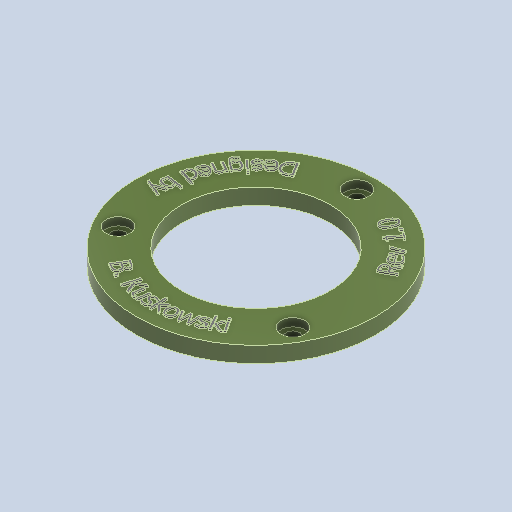
# Autodesk Inventor part: name_plate
Saved by Autodesk Inventor 2025 (Build 290162000, 162)
## iProperties
Created: 2026-08-15
Part Number: name_plate
Material: Ogólny
Document SubType Name: Modeling
Designer: zzapa
Density: 1 g/cm^3
Appearance: Ciemnooliwkowa
Author: zzapa
Autodesk Inventor part; units mm, degrees
ref_plane "YZ Plane" through (0, 0, 0) normal (1, 0, 0) x (0, 1, 0)
ref_plane "XZ Plane" through (0, 0, 0) normal (0, 1, 0) x (-1, 0, 0)
ref_plane "XY Plane" through (0, 0, 0) normal (0, 0, 1) x (1, 0, 0)
sketch "Szkic1" plane through (0, 0, 0) normal (0, 1, 0) x (-1, 0, 0)
  circle A0 centre (0, 0) radius 14
  circle A1 centre (0, 0) radius 22.5
  dimension "d13" = 28
  dimension "d14" = 45
  constraints: 2 centre point, 2 coincident
  measures "d13" diameter of A0
  measures "d14" diameter of A1
extrude "Wyciągnięcie proste1" add sketch "Szkic1" along normal blind 3
sketch "Szkic2" plane through (0, 3, 0) normal (0, 1, 0) x (1, 0, 0)
  line L0 (0, 31.5) -> (0, -31.5) projected
  point P0 (0, 0)
  point P1 (0, 19)
  point P2 (-16.4545, -9.5)
  point P3 (16.4545, -9.5)
  dimension "d4" = 360
  dimension "d15" = 19
  constraints: 1 point on line, 4 other
  measures "d15" distance of point (0, 0) point (0, 19)
hole "Otwór1" at (0, 3, -19) at (-16.4545, 3, 9.5) at (16.4545, 3, 9.5) direction (0, -1, 0) diameter 2.6 end through all counterbore diameter 4.5 counterbore depth 1.5
sketch "Szkic3" plane through (0, 3, 0) normal (0, 1, 0) x (1, 0, 0)
  circle A0 centre (0, 0) radius 14 projected
  circle A1 centre (0, 0) radius 22.5 projected
  circle A2 centre (0, 0) radius 14 projected
  line L0 (0, -14) -> (0, -22.5)
  line L1 (0, 31.5) -> (0, -31.5) projected
  circle A3 centre (0, 0) radius 20
  spline S0 degree 2 poles (-10.7525, 15.0832) (-10.9705, 15.4392) (-11.0329, 16.1888) (-10.8887, 16.4973) knots 0 0 0 1 2 2 2
  spline S1 degree 2 poles (-10.8887, 16.4973) (-10.7669, 16.7428) (-10.412, 17.0761) (-10.096, 17.2696) knots 0 0 0 1 2 2 2
  line L2 (-10.096, 17.2696) -> (-9.4978, 17.636)
  line L3 (-9.4978, 17.636) -> (-7.9058, 15.0369)
  line L4 (-7.9058, 15.0369) -> (-8.4976, 14.6743)
  spline S2 degree 2 poles (-8.4976, 14.6743) (-8.8641, 14.4498) (-9.3483, 14.3039) (-9.555, 14.3105) knots 0 0 0 1 2 2 2
  spline S3 degree 2 poles (-9.555, 14.3105) (-9.9076, 14.3234) (-10.5203, 14.7041) (-10.7525, 15.0832) knots 0 0 0 1 2 2 2
  spline S4 degree 2 poles (-10.3897, 15.2996) (-10.2065, 15.0005) (-9.7492, 14.6984) (-9.4798, 14.6984) knots 0 0 0 1 2 2 2
  spline S5 degree 2 poles (-9.4798, 14.6984) (-9.2905, 14.7014) (-8.9315, 14.8199) (-8.6977, 14.9631) knots 0 0 0 1 2 2 2
  line L5 (-8.6977, 14.9631) -> (-8.4344, 15.1244)
  line L6 (-8.4344, 15.1244) -> (-9.6601, 17.1253)
  line L7 (-9.6601, 17.1253) -> (-9.9234, 16.9641)
  spline S6 degree 2 poles (-9.9234, 16.9641) (-10.1529, 16.8234) (-10.4553, 16.5368) (-10.5358, 16.3514) knots 0 0 0 1 2 2 2
  spline S7 degree 2 poles (-10.5358, 16.3514) (-10.6421, 16.1183) (-10.5755, 15.6029) (-10.3897, 15.2996) knots 0 0 0 1 2 2 2
  spline S8 degree 2 poles (-12.6723, 15.5409) (-12.2444, 15.8838) (-11.3895, 15.7808) (-11.0342, 15.3375) knots 0 0 0 1 2 2 2
  spline S9 degree 2 poles (-11.0342, 15.3375) (-10.6851, 14.9019) (-10.7279, 14.0193) (-11.096, 13.7243) knots 0 0 0 1 2 2 2
  spline S10 degree 2 poles (-11.096, 13.7243) (-11.2618, 13.5914) (-11.5953, 13.4823) (-11.7716, 13.5088) knots 0 0 0 1 2 2 2
  spline S11 degree 2 poles (-11.7716, 13.5088) (-11.9499, 13.5337) (-12.2884, 13.7467) (-12.4598, 13.9607) knots 0 0 0 1 2 2 2
  line L8 (-12.4598, 13.9607) -> (-12.5911, 14.1245)
  line L9 (-12.5911, 14.1245) -> (-11.3557, 15.1147)
  spline S12 degree 2 poles (-11.3557, 15.1147) (-11.6044, 15.425) (-12.1808, 15.5043) (-12.4583, 15.2819) knots 0 0 0 1 2 2 2
  spline S13 degree 2 poles (-12.4583, 15.2819) (-12.5566, 15.2031) (-12.7119, 15.0058) (-12.7612, 14.9094) knots 0 0 0 1 2 2 2
  spline S14 degree 2 poles (-12.7612, 14.9094) (-12.8112, 14.8059) (-12.869, 14.6489) (-12.8809, 14.5887) knots 0 0 0 1 2 2 2
  line L10 (-12.8809, 14.5887) -> (-12.8982, 14.5748)
  line L11 (-12.8982, 14.5748) -> (-13.1608, 14.9024)
  spline S15 degree 2 poles (-13.1608, 14.9024) (-13.1258, 14.9654) (-13.0172, 15.1537) (-12.9694, 15.2205) knots 0 0 0 1 2 2 2
  spline S16 degree 2 poles (-12.9694, 15.2205) (-12.9027, 15.315) (-12.7802, 15.4544) (-12.6723, 15.5409) knots 0 0 0 1 2 2 2
  spline S17 degree 2 poles (-12.1144, 14.1299) (-12.0132, 14.0116) (-11.821, 13.8745) (-11.7249, 13.8533) knots 0 0 0 1 2 2 2
  spline S18 degree 2 poles (-11.7249, 13.8533) (-11.6188, 13.8276) (-11.3978, 13.8876) (-11.2764, 13.9849) knots 0 0 0 1 2 2 2
  spline S19 degree 2 poles (-11.2764, 13.9849) (-11.1569, 14.0806) (-11.0464, 14.2864) (-11.0326, 14.4113) knots 0 0 0 1 2 2 2
  spline S20 degree 2 poles (-11.0326, 14.4113) (-11.0223, 14.5367) (-11.0904, 14.7639) (-11.1719, 14.8853) knots 0 0 0 1 2 2 2
  line L12 (-11.1719, 14.8853) -> (-12.1144, 14.1299)
  spline S21 degree 2 poles (-14.0398, 14.32) (-13.8761, 14.4811) (-13.506, 14.672) (-13.3642, 14.7146) knots 0 0 0 1 2 2 2
  line L13 (-13.3642, 14.7146) -> (-13.061, 14.4065)
  line L14 (-13.061, 14.4065) -> (-13.0751, 14.3926)
  spline S22 degree 2 poles (-13.0751, 14.3926) (-13.138, 14.3861) (-13.2989, 14.3595) (-13.4145, 14.3185) knots 0 0 0 1 2 2 2
  spline S23 degree 2 poles (-13.4145, 14.3185) (-13.5161, 14.2844) (-13.7336, 14.1673) (-13.8234, 14.079) knots 0 0 0 1 2 2 2
  spline S24 degree 2 poles (-13.8234, 14.079) (-13.8885, 14.0148) (-14.0087, 13.8377) (-14.0197, 13.7784) knots 0 0 0 1 2 2 2
  spline S25 degree 2 poles (-14.0197, 13.7784) (-14.0378, 13.6947) (-14.0091, 13.5739) (-13.9329, 13.4965) knots 0 0 0 1 2 2 2
  spline S26 degree 2 poles (-13.9329, 13.4965) (-13.8376, 13.3996) (-13.6332, 13.4032) (-13.4647, 13.5032) knots 0 0 0 1 2 2 2
  spline S27 degree 2 poles (-13.4647, 13.5032) (-13.3998, 13.5429) (-13.1961, 13.674) (-13.1049, 13.7257) knots 0 0 0 1 2 2 2
  spline S28 degree 2 poles (-13.1049, 13.7257) (-12.8646, 13.8547) (-12.4738, 13.7957) (-12.3161, 13.6355) knots 0 0 0 1 2 2 2
  spline S29 degree 2 poles (-12.3161, 13.6355) (-12.0978, 13.4137) (-12.1585, 12.8099) (-12.4331, 12.5396) knots 0 0 0 1 2 2 2
  spline S30 degree 2 poles (-12.4331, 12.5396) (-12.5687, 12.4062) (-12.9092, 12.2028) (-13.0527, 12.162) knots 0 0 0 1 2 2 2
  line L15 (-13.0527, 12.162) -> (-13.3421, 12.456)
  line L16 (-13.3421, 12.456) -> (-13.328, 12.4699)
  spline S31 degree 2 poles (-13.328, 12.4699) (-13.1392, 12.4893) (-12.7869, 12.6455) (-12.6548, 12.7754) knots 0 0 0 1 2 2 2
  spline S32 degree 2 poles (-12.6548, 12.7754) (-12.5193, 12.9088) (-12.4453, 13.2069) (-12.5579, 13.3213) knots 0 0 0 1 2 2 2
  spline S33 degree 2 poles (-12.5579, 13.3213) (-12.6601, 13.4252) (-12.8698, 13.4164) (-13.0242, 13.3268) knots 0 0 0 1 2 2 2
  spline S34 degree 2 poles (-13.0242, 13.3268) (-13.0997, 13.2837) (-13.2822, 13.1664) (-13.384, 13.1043) knots 0 0 0 1 2 2 2
  spline S35 degree 2 poles (-13.384, 13.1043) (-13.6087, 12.9734) (-13.9979, 13.0027) (-14.1764, 13.184) knots 0 0 0 1 2 2 2
  spline S36 degree 2 poles (-14.1764, 13.184) (-14.2803, 13.2896) (-14.3812, 13.5577) (-14.3678, 13.706) knots 0 0 0 1 2 2 2
  spline S37 degree 2 poles (-14.3678, 13.706) (-14.3526, 13.8631) (-14.2071, 14.1554) (-14.0398, 14.32) knots 0 0 0 1 2 2 2
  line L17 (-15.1279, 13.0838) -> (-14.873, 13.3728)
  line L18 (-14.873, 13.3728) -> (-13.1575, 11.86)
  line L19 (-13.1575, 11.86) -> (-13.4124, 11.571)
  line L20 (-13.4124, 11.571) -> (-15.1279, 13.0838)
  line L21 (-13.1451, 11.299) -> (-12.8559, 11.6269)
  line L22 (-12.8559, 11.6269) -> (-12.5558, 11.3622)
  line L23 (-12.5558, 11.3622) -> (-12.8449, 11.0343)
  line L24 (-12.8449, 11.0343) -> (-13.1451, 11.299)
  spline S38 degree 2 poles (-15.8473, 12.8162) (-15.8848, 12.7949) (-16.0184, 12.7066) (-16.0938, 12.6427) knots 0 0 0 1 2 2 2
  spline S39 degree 2 poles (-16.0938, 12.6427) (-16.1791, 12.5738) (-16.3127, 12.4485) (-16.3762, 12.3633) knots 0 0 0 1 2 2 2
  spline S40 degree 2 poles (-16.3762, 12.3633) (-16.4825, 12.2208) (-16.555, 11.9667) (-16.529, 11.861) knots 0 0 0 1 2 2 2
  spline S41 degree 2 poles (-16.529, 11.861) (-16.5015, 11.7574) (-16.3564, 11.5844) (-16.2435, 11.5002) knots 0 0 0 1 2 2 2
  line L25 (-16.2435, 11.5002) -> (-16.0831, 11.3805)
  spline S42 degree 2 poles (-16.0831, 11.3805) (-16.099, 11.5865) (-16.0232, 11.9029) (-15.8888, 12.083) knots 0 0 0 1 2 2 2
  spline S43 degree 2 poles (-15.8888, 12.083) (-15.6555, 12.3959) (-14.9141, 12.419) (-14.4765, 12.0927) knots 0 0 0 1 2 2 2
  spline S44 degree 2 poles (-14.4765, 12.0927) (-14.2488, 11.9228) (-13.9924, 11.5312) (-13.9474, 11.3313) knots 0 0 0 1 2 2 2
  spline S45 degree 2 poles (-13.9474, 11.3313) (-13.9074, 11.1412) (-13.9899, 10.7621) (-14.1021, 10.6116) knots 0 0 0 1 2 2 2
  spline S46 degree 2 poles (-14.1021, 10.6116) (-14.2085, 10.4691) (-14.4309, 10.3114) (-14.5705, 10.2522) knots 0 0 0 1 2 2 2
  line L26 (-14.5705, 10.2522) -> (-14.5066, 10.1768)
  line L27 (-14.5066, 10.1768) -> (-14.7237, 9.8858)
  line L28 (-14.7237, 9.8858) -> (-16.3472, 11.0968)
  spline S47 degree 2 poles (-16.3472, 11.0968) (-16.8144, 11.4453) (-16.9472, 12.1761) (-16.6356, 12.5939) knots 0 0 0 1 2 2 2
  spline S48 degree 2 poles (-16.6356, 12.5939) (-16.5352, 12.7285) (-16.2819, 12.9771) (-16.1562, 13.0713) knots 0 0 0 1 2 2 2
  line L29 (-16.1562, 13.0713) -> (-15.8355, 12.8321)
  line L30 (-15.8355, 12.8321) -> (-15.8473, 12.8162)
  line L31 (-15.8297, 11.1915) -> (-14.8219, 10.4398)
  spline S49 degree 2 poles (-14.8219, 10.4398) (-14.6809, 10.5133) (-14.4886, 10.6719) (-14.4162, 10.7689) knots 0 0 0 1 2 2 2
  spline S50 degree 2 poles (-14.4162, 10.7689) (-14.242, 11.0025) (-14.3856, 11.5287) (-14.7083, 11.7695) knots 0 0 0 1 2 2 2
  spline S51 degree 2 poles (-14.7083, 11.7695) (-15.0132, 11.9969) (-15.4841, 12.0307) (-15.6554, 11.8011) knots 0 0 0 1 2 2 2
  spline S52 degree 2 poles (-15.6554, 11.8011) (-15.7455, 11.6803) (-15.8395, 11.356) (-15.8297, 11.1915) knots 0 0 0 1 2 2 2
  line L32 (-17.7638, 9.2342) -> (-17.5707, 9.5677)
  line L33 (-17.5707, 9.5677) -> (-16.442, 8.9144)
  spline S53 degree 2 poles (-16.442, 8.9144) (-16.3052, 8.8352) (-16.0552, 8.7248) (-15.9624, 8.7224) knots 0 0 0 1 2 2 2
  spline S54 degree 2 poles (-15.9624, 8.7224) (-15.864, 8.7197) (-15.7072, 8.823) (-15.6354, 8.947) knots 0 0 0 1 2 2 2
  spline S55 degree 2 poles (-15.6354, 8.947) (-15.5637, 9.071) (-15.544, 9.4106) (-15.5779, 9.5986) knots 0 0 0 1 2 2 2
  line L34 (-15.5779, 9.5986) -> (-17.0572, 10.4549)
  line L35 (-17.0572, 10.4549) -> (-16.8642, 10.7884)
  line L36 (-16.8642, 10.7884) -> (-14.8847, 9.6426)
  line L37 (-14.8847, 9.6426) -> (-15.0777, 9.3091)
  line L38 (-15.0777, 9.3091) -> (-15.2979, 9.4366)
  spline S56 degree 2 poles (-15.2979, 9.4366) (-15.2498, 9.209) (-15.2758, 8.8387) (-15.3698, 8.6762) knots 0 0 0 1 2 2 2
  spline S57 degree 2 poles (-15.3698, 8.6762) (-15.5381, 8.3855) (-16.1134, 8.279) (-16.479, 8.4906) knots 0 0 0 1 2 2 2
  line L39 (-16.479, 8.4906) -> (-17.7638, 9.2342)
  spline S58 degree 2 poles (-18.4477, 7.8607) (-18.2285, 8.3633) (-17.4238, 8.6699) (-16.903, 8.4428) knots 0 0 0 1 2 2 2
  spline S59 degree 2 poles (-16.903, 8.4428) (-16.3914, 8.2196) (-16.0186, 7.4184) (-16.2072, 6.986) knots 0 0 0 1 2 2 2
  spline S60 degree 2 poles (-16.2072, 6.986) (-16.2921, 6.7913) (-16.5366, 6.5395) (-16.705, 6.4809) knots 0 0 0 1 2 2 2
  spline S61 degree 2 poles (-16.705, 6.4809) (-16.8744, 6.42) (-17.2731, 6.4511) (-17.5244, 6.5607) knots 0 0 0 1 2 2 2
  line L40 (-17.5244, 6.5607) -> (-17.7169, 6.6446)
  line L41 (-17.7169, 6.6446) -> (-17.0839, 8.0959)
  spline S62 degree 2 poles (-17.0839, 8.0959) (-17.4485, 8.2549) (-17.9956, 8.0569) (-18.1378, 7.7309) knots 0 0 0 1 2 2 2
  spline S63 degree 2 poles (-18.1378, 7.7309) (-18.1881, 7.6155) (-18.2338, 7.3686) (-18.2325, 7.2603) knots 0 0 0 1 2 2 2
  spline S64 degree 2 poles (-18.2325, 7.2603) (-18.2287, 7.1454) (-18.2068, 6.9796) (-18.1893, 6.9207) knots 0 0 0 1 2 2 2
  line L42 (-18.1893, 6.9207) -> (-18.1982, 6.9004)
  line L43 (-18.1982, 6.9004) -> (-18.5831, 7.0682)
  spline S65 degree 2 poles (-18.5831, 7.0682) (-18.5813, 7.1402) (-18.5728, 7.3575) (-18.5616, 7.4388) knots 0 0 0 1 2 2 2
  spline S66 degree 2 poles (-18.5616, 7.4388) (-18.5466, 7.5535) (-18.5029, 7.7339) (-18.4477, 7.8607) knots 0 0 0 1 2 2 2
  spline S67 degree 2 poles (-17.2974, 6.8713) (-17.1527, 6.8136) (-16.9188, 6.7816) (-16.8239, 6.8076) knots 0 0 0 1 2 2 2
  spline S68 degree 2 poles (-16.8239, 6.8076) (-16.718, 6.8342) (-16.5503, 6.9901) (-16.4881, 7.1327) knots 0 0 0 1 2 2 2
  spline S69 degree 2 poles (-16.4881, 7.1327) (-16.4269, 7.2731) (-16.4247, 7.5066) (-16.4707, 7.6237) knots 0 0 0 1 2 2 2
  spline S70 degree 2 poles (-16.4707, 7.6237) (-16.5199, 7.7395) (-16.6859, 7.9088) (-16.8145, 7.9784) knots 0 0 0 1 2 2 2
  line L44 (-16.8145, 7.9784) -> (-17.2974, 6.8713)
  line L45 (-19.3752, 5.0374) -> (-19.2619, 5.4058)
  line L46 (-19.2619, 5.4058) -> (-19.04, 5.3375)
  spline S71 degree 2 poles (-19.04, 5.3375) (-19.0847, 5.4443) (-19.1407, 5.5985) (-19.1547, 5.6958) knots 0 0 0 1 2 2 2
  spline S72 degree 2 poles (-19.1547, 5.6958) (-19.1685, 5.7853) (-19.1571, 5.9653) (-19.123, 6.0762) knots 0 0 0 1 2 2 2
  spline S73 degree 2 poles (-19.123, 6.0762) (-19.0678, 6.2557) (-18.8261, 6.5121) (-18.6494, 6.5741) knots 0 0 0 1 2 2 2
  spline S74 degree 2 poles (-18.6494, 6.5741) (-18.4728, 6.6361) (-18.0115, 6.6234) (-17.7353, 6.5385) knots 0 0 0 1 2 2 2
  spline S75 degree 2 poles (-17.7353, 6.5385) (-17.4472, 6.4499) (-17.0727, 6.172) (-16.9545, 5.9935) knots 0 0 0 1 2 2 2
  spline S76 degree 2 poles (-16.9545, 5.9935) (-16.8498, 5.8295) (-16.7907, 5.4418) (-16.8481, 5.2553) knots 0 0 0 1 2 2 2
  spline S77 degree 2 poles (-16.8481, 5.2553) (-16.8982, 5.0924) (-17.0461, 4.8717) (-17.1631, 4.7604) knots 0 0 0 1 2 2 2
  line L47 (-17.1631, 4.7604) -> (-16.2187, 4.47)
  line L48 (-16.2187, 4.47) -> (-16.3319, 4.1017)
  line L49 (-16.3319, 4.1017) -> (-19.3752, 5.0374)
  line L50 (-18.7307, 5.2424) -> (-17.4676, 4.854)
  spline S78 degree 2 poles (-17.4676, 4.854) (-17.3594, 4.9707) (-17.243, 5.1726) (-17.2046, 5.2977) knots 0 0 0 1 2 2 2
  spline S79 degree 2 poles (-17.2046, 5.2977) (-17.1175, 5.5811) (-17.4437, 6.0328) (-17.8451, 6.1562) knots 0 0 0 1 2 2 2
  spline S80 degree 2 poles (-17.8451, 6.1562) (-18.2323, 6.2753) (-18.7162, 6.1553) (-18.7997, 5.8838) knots 0 0 0 1 2 2 2
  spline S81 degree 2 poles (-18.7997, 5.8838) (-18.844, 5.7398) (-18.8018, 5.4064) (-18.7307, 5.2424) knots 0 0 0 1 2 2 2
  spline S82 degree 2 poles (-18.8116, 1.1694) (-19.3684, 1.235) (-19.9844, 1.8546) (-19.9365, 2.2618) knots 0 0 0 1 2 2 2
  spline S83 degree 2 poles (-19.9365, 2.2618) (-19.9148, 2.4458) (-19.7932, 2.6976) (-19.6997, 2.8159) knots 0 0 0 1 2 2 2
  line L51 (-19.6997, 2.8159) -> (-19.8023, 2.8529)
  line L52 (-19.8023, 2.8529) -> (-19.7601, 3.211)
  line L53 (-19.7601, 3.211) -> (-16.5981, 2.8389)
  line L54 (-16.5981, 2.8389) -> (-16.6431, 2.4562)
  line L55 (-16.6431, 2.4562) -> (-17.7716, 2.589)
  spline S84 degree 2 poles (-17.7716, 2.589) (-17.6586, 2.429) (-17.5264, 2.0727) (-17.5515, 1.8593) knots 0 0 0 1 2 2 2
  spline S85 degree 2 poles (-17.5515, 1.8593) (-17.5969, 1.4741) (-18.2646, 1.1051) (-18.8116, 1.1694) knots 0 0 0 1 2 2 2
  spline S86 degree 2 poles (-18.7945, 1.5679) (-18.3873, 1.5199) (-17.9362, 1.718) (-17.9039, 1.9928) knots 0 0 0 1 2 2 2
  spline S87 degree 2 poles (-17.9039, 1.9928) (-17.8857, 2.1473) (-17.9954, 2.4835) (-18.0929, 2.6268) knots 0 0 0 1 2 2 2
  line L56 (-18.0929, 2.6268) -> (-19.3955, 2.7801)
  spline S88 degree 2 poles (-19.3955, 2.7801) (-19.4837, 2.6438) (-19.5688, 2.4275) (-19.5844, 2.295) knots 0 0 0 1 2 2 2
  spline S89 degree 2 poles (-19.5844, 2.295) (-19.6188, 2.0031) (-19.2435, 1.6207) (-18.7945, 1.5679) knots 0 0 0 1 2 2 2
  line L57 (-17.7197, -0.9043) -> (-20.8403, 0.3482)
  line L58 (-20.8403, 0.3482) -> (-20.8374, 0.7607)
  line L59 (-20.8374, 0.7607) -> (-19.8869, 0.3438)
  line L60 (-19.8869, 0.3438) -> (-17.7049, 1.1581)
  line L61 (-17.7049, 1.1581) -> (-17.7079, 0.7432)
  line L62 (-17.7079, 0.7432) -> (-19.4068, 0.1304)
  line L63 (-19.4068, 0.1304) -> (-17.7168, -0.5041)
  line L64 (-17.7168, -0.5041) -> (-17.7197, -0.9043)
  spline S90 degree 2 poles (-8.8291, -16.9346) (-8.946, -17.1294) (-9.2735, -17.3391) (-9.4548, -17.3629) knots 0 0 0 1 2 2 2
  spline S91 degree 2 poles (-9.4548, -17.3629) (-9.6717, -17.3883) (-10.0669, -17.2837) (-10.3338, -17.1236) knots 0 0 0 1 2 2 2
  line L65 (-10.3338, -17.1236) -> (-11.0836, -16.6737)
  line L66 (-11.0836, -16.6737) -> (-9.5155, -14.06)
  line L67 (-9.5155, -14.06) -> (-8.8229, -14.4755)
  spline S92 degree 2 poles (-8.8229, -14.4755) (-8.5433, -14.6433) (-8.2853, -14.847) (-8.2001, -14.9932) knots 0 0 0 1 2 2 2
  spline S93 degree 2 poles (-8.2001, -14.9932) (-8.1027, -15.1524) (-8.1196, -15.4735) (-8.2188, -15.6387) knots 0 0 0 1 2 2 2
  spline S94 degree 2 poles (-8.2188, -15.6387) (-8.3293, -15.823) (-8.6995, -15.9984) (-8.9207, -15.9781) knots 0 0 0 1 2 2 2
  line L68 (-8.9207, -15.9781) -> (-8.9283, -15.9908)
  spline S95 degree 2 poles (-8.9283, -15.9908) (-8.7334, -16.1941) (-8.6792, -16.6846) (-8.8291, -16.9346) knots 0 0 0 1 2 2 2
  spline S96 degree 2 poles (-9.2002, -16.7321) (-9.1113, -16.5838) (-9.0816, -16.3424) (-9.168, -16.1984) knots 0 0 0 1 2 2 2
  spline S97 degree 2 poles (-9.168, -16.1984) (-9.2252, -16.1064) (-9.4048, -15.9641) (-9.5849, -15.8561) knots 0 0 0 1 2 2 2
  line L69 (-9.5849, -15.8561) -> (-9.9788, -15.6197)
  line L70 (-9.9788, -15.6197) -> (-10.5583, -16.5856)
  line L71 (-10.5583, -16.5856) -> (-10.2766, -16.7546)
  spline S98 degree 2 poles (-10.2766, -16.7546) (-10.0478, -16.8918) (-9.7598, -17.007) (-9.6175, -17.0003) knots 0 0 0 1 2 2 2
  spline S99 degree 2 poles (-9.6175, -17.0003) (-9.4781, -16.9888) (-9.2828, -16.8698) (-9.2002, -16.7321) knots 0 0 0 1 2 2 2
  spline S100 degree 2 poles (-8.6102, -15.4702) (-8.5543, -15.377) (-8.5339, -15.1991) (-8.5797, -15.1169) knots 0 0 0 1 2 2 2
  spline S101 degree 2 poles (-8.5797, -15.1169) (-8.6365, -15.0194) (-8.8292, -14.875) (-9.0135, -14.7645) knots 0 0 0 1 2 2 2
  line L72 (-9.0135, -14.7645) -> (-9.346, -14.5649)
  line L73 (-9.346, -14.5649) -> (-9.8047, -15.3296)
  line L74 (-9.8047, -15.3296) -> (-9.4108, -15.5659)
  spline S102 degree 2 poles (-9.4108, -15.5659) (-9.2477, -15.6638) (-9.0727, -15.7226) (-8.9584, -15.7193) knots 0 0 0 1 2 2 2
  spline S103 degree 2 poles (-8.9584, -15.7193) (-8.8474, -15.7167) (-8.6839, -15.593) (-8.6102, -15.4702) knots 0 0 0 1 2 2 2
  line L75 (-8.4266, -18.1397) -> (-8.8676, -17.9284)
  line L76 (-8.8676, -17.9284) -> (-8.6157, -17.4027)
  line L77 (-8.6157, -17.4027) -> (-8.1747, -17.6141)
  line L78 (-8.1747, -17.6141) -> (-8.4266, -18.1397)
  line L79 (-4.4403, -19.5441) -> (-4.9447, -19.3945)
  line L80 (-4.9447, -19.3945) -> (-5.6096, -17.7185)
  line L81 (-5.6096, -17.7185) -> (-5.837, -17.8598)
  line L82 (-5.837, -17.8598) -> (-6.1832, -19.0273)
  line L83 (-6.1832, -19.0273) -> (-6.5716, -18.9121)
  line L84 (-6.5716, -18.9121) -> (-5.705, -15.9899)
  line L85 (-5.705, -15.9899) -> (-5.3167, -16.105)
  line L86 (-5.3167, -16.105) -> (-5.7148, -17.4478)
  line L87 (-5.7148, -17.4478) -> (-4.1184, -16.4604)
  line L88 (-4.1184, -16.4604) -> (-3.6448, -16.6008)
  line L89 (-3.6448, -16.6008) -> (-5.2418, -17.5468)
  line L90 (-5.2418, -17.5468) -> (-4.4403, -19.5441)
  line L91 (-2.4749, -19.8662) -> (-2.8548, -19.8016)
  line L92 (-2.8548, -19.8016) -> (-2.8126, -19.5532)
  spline S104 degree 2 poles (-2.8126, -19.5532) (-3.014, -19.6768) (-3.355, -19.7817) (-3.5498, -19.7486) knots 0 0 0 1 2 2 2
  spline S105 degree 2 poles (-3.5498, -19.7486) (-3.6959, -19.7238) (-3.9399, -19.5821) (-4.0171, -19.4612) knots 0 0 0 1 2 2 2
  spline S106 degree 2 poles (-4.0171, -19.4612) (-4.0967, -19.34) (-4.1496, -19.0028) (-4.1107, -18.7739) knots 0 0 0 1 2 2 2
  line L93 (-4.1107, -18.7739) -> (-3.862, -17.3104)
  line L94 (-3.862, -17.3104) -> (-3.4821, -17.3749)
  line L95 (-3.4821, -17.3749) -> (-3.7006, -18.6607)
  spline S107 degree 2 poles (-3.7006, -18.6607) (-3.7313, -18.8409) (-3.7446, -19.0816) (-3.7133, -19.1772) knots 0 0 0 1 2 2 2
  spline S108 degree 2 poles (-3.7133, -19.1772) (-3.6819, -19.2727) (-3.5373, -19.3799) (-3.3887, -19.4052) knots 0 0 0 1 2 2 2
  spline S109 degree 2 poles (-3.3887, -19.4052) (-3.2499, -19.4288) (-2.9089, -19.3239) (-2.7579, -19.2318) knots 0 0 0 1 2 2 2
  line L96 (-2.7579, -19.2318) -> (-2.4715, -17.5467)
  line L97 (-2.4715, -17.5467) -> (-2.0916, -17.6113)
  line L98 (-2.0916, -17.6113) -> (-2.4749, -19.8662)
  spline S110 degree 2 poles (-1.307, -20.0117) (-1.5363, -19.9972) (-1.9254, -19.8488) (-2.0516, -19.7715) knots 0 0 0 1 2 2 2
  line L99 (-2.0516, -19.7715) -> (-2.0243, -19.3401)
  line L100 (-2.0243, -19.3401) -> (-2.0046, -19.3413)
  spline S111 degree 2 poles (-2.0046, -19.3413) (-1.9578, -19.3839) (-1.8306, -19.486) (-1.7229, -19.5448) knots 0 0 0 1 2 2 2
  spline S112 degree 2 poles (-1.7229, -19.5448) (-1.6298, -19.5978) (-1.3975, -19.6818) (-1.2718, -19.6898) knots 0 0 0 1 2 2 2
  spline S113 degree 2 poles (-1.2718, -19.6898) (-1.1806, -19.6955) (-0.9684, -19.6669) (-0.9169, -19.6355) knots 0 0 0 1 2 2 2
  spline S114 degree 2 poles (-0.9169, -19.6355) (-0.8424, -19.5932) (-0.7716, -19.4913) (-0.7648, -19.3828) knots 0 0 0 1 2 2 2
  spline S115 degree 2 poles (-0.7648, -19.3828) (-0.7562, -19.2472) (-0.8952, -19.0974) (-1.082, -19.0385) knots 0 0 0 1 2 2 2
  spline S116 degree 2 poles (-1.082, -19.0385) (-1.1549, -19.0165) (-1.3884, -18.9522) (-1.4877, -18.9187) knots 0 0 0 1 2 2 2
  spline S117 degree 2 poles (-1.4877, -18.9187) (-1.7442, -18.8257) (-1.9608, -18.4952) (-1.9466, -18.2709) knots 0 0 0 1 2 2 2
  spline S118 degree 2 poles (-1.9466, -18.2709) (-1.9269, -17.9603) (-1.4365, -17.6028) (-1.0519, -17.6272) knots 0 0 0 1 2 2 2
  spline S119 degree 2 poles (-1.0519, -17.6272) (-0.8621, -17.6392) (-0.4835, -17.7573) (-0.3574, -17.837) knots 0 0 0 1 2 2 2
  line L101 (-0.3574, -17.837) -> (-0.3835, -18.2487)
  line L102 (-0.3835, -18.2487) -> (-0.4032, -18.2475)
  spline S120 degree 2 poles (-0.4032, -18.2475) (-0.5436, -18.1198) (-0.8949, -17.9614) (-1.0798, -17.9496) knots 0 0 0 1 2 2 2
  spline S121 degree 2 poles (-1.0798, -17.9496) (-1.2696, -17.9376) (-1.5411, -18.0813) (-1.5512, -18.2415) knots 0 0 0 1 2 2 2
  spline S122 degree 2 poles (-1.5512, -18.2415) (-1.5604, -18.3869) (-1.414, -18.5373) (-1.2443, -18.5926) knots 0 0 0 1 2 2 2
  spline S123 degree 2 poles (-1.2443, -18.5926) (-1.1619, -18.6201) (-0.9527, -18.6779) (-0.8386, -18.7124) knots 0 0 0 1 2 2 2
  spline S124 degree 2 poles (-0.8386, -18.7124) (-0.5912, -18.7924) (-0.3534, -19.102) (-0.3695, -19.3559) knots 0 0 0 1 2 2 2
  spline S125 degree 2 poles (-0.3695, -19.3559) (-0.3789, -19.5038) (-0.5113, -19.7578) (-0.6308, -19.8467) knots 0 0 0 1 2 2 2
  spline S126 degree 2 poles (-0.6308, -19.8467) (-0.758, -19.9401) (-1.0729, -20.0266) (-1.307, -20.0117) knots 0 0 0 1 2 2 2
  line L103 (1.8398, -19.9472) -> (1.3338, -19.9652)
  line L104 (1.3338, -19.9652) -> (0.4454, -18.892)
  line L105 (0.4454, -18.892) -> (0.2976, -19.0456)
  line L106 (0.2976, -19.0456) -> (0.3316, -20.0008)
  line L107 (0.3316, -20.0008) -> (-0.0535, -20.0145)
  line L108 (-0.0535, -20.0145) -> (-0.1666, -16.8327)
  line L109 (-0.1666, -16.8327) -> (0.2185, -16.819)
  line L110 (0.2185, -16.819) -> (0.2846, -18.6802)
  line L111 (0.2846, -18.6802) -> (1.1538, -17.6829)
  line L112 (1.1538, -17.6829) -> (1.6326, -17.6659)
  line L113 (1.6326, -17.6659) -> (0.7286, -18.6546)
  line L114 (0.7286, -18.6546) -> (1.8398, -19.9472)
  spline S127 degree 2 poles (3.7255, -18.5129) (3.8087, -19.0849) (3.3494, -19.7882) (2.8899, -19.855) knots 0 0 0 1 2 2 2
  spline S128 degree 2 poles (2.8899, -19.855) (2.4182, -19.9236) (1.7844, -19.3594) (1.7041, -18.807) knots 0 0 0 1 2 2 2
  spline S129 degree 2 poles (1.7041, -18.807) (1.6216, -18.2399) (2.0875, -17.5306) (2.5421, -17.4645) knots 0 0 0 1 2 2 2
  spline S130 degree 2 poles (2.5421, -17.4645) (3.0016, -17.3976) (3.6426, -17.9434) (3.7255, -18.5129) knots 0 0 0 1 2 2 2
  spline S131 degree 2 poles (3.332, -18.5701) (3.268, -18.1302) (2.8855, -17.749) (2.5898, -17.792) knots 0 0 0 1 2 2 2
  spline S132 degree 2 poles (2.5898, -17.792) (2.294, -17.8351) (2.0336, -18.3098) (2.0976, -18.7497) knots 0 0 0 1 2 2 2
  spline S133 degree 2 poles (2.0976, -18.7497) (2.1598, -19.1775) (2.5465, -19.5705) (2.8422, -19.5275) knots 0 0 0 1 2 2 2
  spline S134 degree 2 poles (2.8422, -19.5275) (3.1356, -19.4848) (3.3953, -19.0052) (3.332, -18.5701) knots 0 0 0 1 2 2 2
  line L115 (6.3136, -16.6168) -> (6.3852, -18.9754)
  line L116 (6.3852, -18.9754) -> (6.0433, -19.0733)
  line L117 (6.0433, -19.0733) -> (5.0212, -17.5315)
  line L118 (5.0212, -17.5315) -> (4.9723, -19.38)
  line L119 (4.9723, -19.38) -> (4.6328, -19.4772)
  line L120 (4.6328, -19.4772) -> (3.4404, -17.4395)
  line L121 (3.4404, -17.4395) -> (3.8251, -17.3293)
  line L122 (3.8251, -17.3293) -> (4.702, -18.9204)
  line L123 (4.702, -18.9204) -> (4.7345, -17.0689)
  line L124 (4.7345, -17.0689) -> (5.0409, -16.9812)
  line L125 (5.0409, -16.9812) -> (6.0626, -18.5308)
  line L126 (6.0626, -18.5308) -> (5.9408, -16.7235)
  line L127 (5.9408, -16.7235) -> (6.3136, -16.6168)
  spline S135 degree 2 poles (7.8328, -18.4614) (7.6216, -18.5516) (7.2073, -18.594) (7.0598, -18.5817) knots 0 0 0 1 2 2 2
  line L128 (7.0598, -18.5817) -> (6.8902, -18.1841)
  line L129 (6.8902, -18.1841) -> (6.9083, -18.1764)
  spline S136 degree 2 poles (6.9083, -18.1764) (6.9693, -18.1934) (7.1288, -18.2274) (7.2514, -18.2315) knots 0 0 0 1 2 2 2
  spline S137 degree 2 poles (7.2514, -18.2315) (7.3584, -18.2368) (7.6037, -18.2074) (7.7195, -18.158) knots 0 0 0 1 2 2 2
  spline S138 degree 2 poles (7.7195, -18.158) (7.8036, -18.1221) (7.9802, -18.0011) (8.0121, -17.95) knots 0 0 0 1 2 2 2
  spline S139 degree 2 poles (8.0121, -17.95) (8.0596, -17.8787) (8.077, -17.7558) (8.0343, -17.6558) knots 0 0 0 1 2 2 2
  spline S140 degree 2 poles (8.0343, -17.6558) (7.981, -17.5309) (7.7895, -17.4595) (7.5961, -17.491) knots 0 0 0 1 2 2 2
  spline S141 degree 2 poles (7.5961, -17.491) (7.5212, -17.5041) (7.2837, -17.5517) (7.1799, -17.5665) knots 0 0 0 1 2 2 2
  spline S142 degree 2 poles (7.1799, -17.5665) (6.909, -17.5988) (6.5669, -17.401) (6.4787, -17.1942) knots 0 0 0 1 2 2 2
  spline S143 degree 2 poles (6.4787, -17.1942) (6.3566, -16.908) (6.6338, -16.3681) (6.9883, -16.2169) knots 0 0 0 1 2 2 2
  spline S144 degree 2 poles (6.9883, -16.2169) (7.1632, -16.1423) (7.5545, -16.0775) (7.703, -16.092) knots 0 0 0 1 2 2 2
  line L130 (7.703, -16.092) -> (7.8648, -16.4714)
  line L131 (7.8648, -16.4714) -> (7.8466, -16.4792)
  spline S145 degree 2 poles (7.8466, -16.4792) (7.6638, -16.4282) (7.2788, -16.4448) (7.1084, -16.5175) knots 0 0 0 1 2 2 2
  spline S146 degree 2 poles (7.1084, -16.5175) (6.9335, -16.5921) (6.7556, -16.8425) (6.8186, -16.9902) knots 0 0 0 1 2 2 2
  spline S147 degree 2 poles (6.8186, -16.9902) (6.8758, -17.1242) (7.0742, -17.1926) (7.2506, -17.1657) knots 0 0 0 1 2 2 2
  spline S148 degree 2 poles (7.2506, -17.1657) (7.3366, -17.1532) (7.5494, -17.1108) (7.6669, -17.0902) knots 0 0 0 1 2 2 2
  spline S149 degree 2 poles (7.6669, -17.0902) (7.9238, -17.0504) (8.2754, -17.22) (8.3752, -17.454) knots 0 0 0 1 2 2 2
  spline S150 degree 2 poles (8.3752, -17.454) (8.4334, -17.5903) (8.4293, -17.8767) (8.3626, -18.0099) knots 0 0 0 1 2 2 2
  spline S151 degree 2 poles (8.3626, -18.0099) (8.291, -18.1505) (8.0487, -18.3694) (7.8328, -18.4614) knots 0 0 0 1 2 2 2
  line L132 (10.6144, -16.9885) -> (10.1706, -17.2322)
  line L133 (10.1706, -17.2322) -> (8.8944, -16.6732)
  line L134 (8.8944, -16.6732) -> (8.8315, -16.8768)
  line L135 (8.8315, -16.8768) -> (9.2915, -17.7147)
  line L136 (9.2915, -17.7147) -> (8.9537, -17.9002)
  line L137 (8.9537, -17.9002) -> (7.4216, -15.1092)
  line L138 (7.4216, -15.1092) -> (7.7594, -14.9237)
  line L139 (7.7594, -14.9237) -> (8.6556, -16.5563)
  line L140 (8.6556, -16.5563) -> (8.9834, -15.2747)
  line L141 (8.9834, -15.2747) -> (9.4034, -15.0441)
  line L142 (9.4034, -15.0441) -> (9.0406, -16.3337)
  line L143 (9.0406, -16.3337) -> (10.6144, -16.9885)
  line L144 (11.09, -16.6448) -> (10.7673, -16.8553)
  line L145 (10.7673, -16.8553) -> (9.5175, -14.9398)
  line L146 (9.5175, -14.9398) -> (9.8402, -14.7292)
  line L147 (9.8402, -14.7292) -> (11.09, -16.6448)
  line L148 (9.6551, -14.3958) -> (9.289, -14.6347)
  line L149 (9.289, -14.6347) -> (9.0703, -14.2996)
  line L150 (9.0703, -14.2996) -> (9.4365, -14.0607)
  line L151 (9.4365, -14.0607) -> (9.6551, -14.3958)
  line L152 (16.9016, 10.7798) -> (17.1536, 10.318)
  line L153 (17.1536, 10.318) -> (16.5504, 8.8914)
  line L154 (16.5504, 8.8914) -> (16.7729, 8.4838)
  line L155 (16.7729, 8.4838) -> (17.8375, 9.0647)
  line L156 (17.8375, 9.0647) -> (18.0315, 8.7091)
  line L157 (18.0315, 8.7091) -> (15.3559, 7.2492)
  line L158 (15.3559, 7.2492) -> (14.9797, 7.9387)
  spline S152 degree 2 poles (14.9797, 7.9387) (14.8542, 8.1685) (14.7349, 8.5058) (14.7491, 8.6964) knots 0 0 0 1 2 2 2
  spline S153 degree 2 poles (14.7491, 8.6964) (14.7633, 8.887) (14.9586, 9.2046) (15.1689, 9.3194) knots 0 0 0 1 2 2 2
  spline S154 degree 2 poles (15.1689, 9.3194) (15.4616, 9.4791) (16.0217, 9.3964) (16.2567, 9.1926) knots 0 0 0 1 2 2 2
  line L159 (16.2567, 9.1926) -> (16.9016, 10.7798)
  spline S155 degree 2 poles (15.3994, 8.964) (15.2823, 8.9001) (15.1473, 8.7195) (15.1361, 8.6009) knots 0 0 0 1 2 2 2
  spline S156 degree 2 poles (15.1361, 8.6009) (15.1276, 8.4978) (15.1964, 8.2736) (15.2769, 8.1262) knots 0 0 0 1 2 2 2
  line L160 (15.2769, 8.1262) -> (15.4697, 7.7728)
  line L161 (15.4697, 7.7728) -> (16.4758, 8.3217)
  line L162 (16.4758, 8.3217) -> (16.3054, 8.634)
  spline S157 degree 2 poles (16.3054, 8.634) (16.2214, 8.7879) (16.0335, 9.0033) (15.9028, 9.0418) knots 0 0 0 1 2 2 2
  spline S158 degree 2 poles (15.9028, 9.0418) (15.7865, 9.0796) (15.5382, 9.0397) (15.3994, 8.964) knots 0 0 0 1 2 2 2
  spline S159 degree 2 poles (16.2272, 11.7807) (16.5456, 11.3342) (16.3948, 10.4865) (15.9323, 10.1566) knots 0 0 0 1 2 2 2
  spline S160 degree 2 poles (15.9323, 10.1566) (15.4778, 9.8325) (14.5989, 9.9247) (14.325, 10.3088) knots 0 0 0 1 2 2 2
  spline S161 degree 2 poles (14.325, 10.3088) (14.2017, 10.4817) (14.1115, 10.8209) (14.1478, 10.9955) knots 0 0 0 1 2 2 2
  spline S162 degree 2 poles (14.1478, 10.9955) (14.1826, 11.172) (14.4143, 11.498) (14.6375, 11.6572) knots 0 0 0 1 2 2 2
  line L163 (14.6375, 11.6572) -> (14.8085, 11.7791)
  line L164 (14.8085, 11.7791) -> (15.7278, 10.4901)
  spline S163 degree 2 poles (15.7278, 10.4901) (16.0515, 10.721) (16.1631, 11.292) (15.9566, 11.5816) knots 0 0 0 1 2 2 2
  spline S164 degree 2 poles (15.9566, 11.5816) (15.8834, 11.6842) (15.6952, 11.8503) (15.6016, 11.9049) knots 0 0 0 1 2 2 2
  spline S165 degree 2 poles (15.6016, 11.9049) (15.5012, 11.9607) (15.3476, 12.0271) (15.2882, 12.0424) knots 0 0 0 1 2 2 2
  line L165 (15.2882, 12.0424) -> (15.2753, 12.0605)
  line L166 (15.2753, 12.0605) -> (15.6171, 12.3043)
  spline S166 degree 2 poles (15.6171, 12.3043) (15.678, 12.2658) (15.8599, 12.1468) (15.9239, 12.0953) knots 0 0 0 1 2 2 2
  spline S167 degree 2 poles (15.9239, 12.0953) (16.0146, 12.0235) (16.1469, 11.8933) (16.2272, 11.7807) knots 0 0 0 1 2 2 2
  spline S168 degree 2 poles (14.7871, 11.3028) (14.6633, 11.2084) (14.5156, 11.0242) (14.4891, 10.9295) knots 0 0 0 1 2 2 2
  spline S169 degree 2 poles (14.4891, 10.9295) (14.4575, 10.825) (14.505, 10.601) (14.5953, 10.4743) knots 0 0 0 1 2 2 2
  spline S170 degree 2 poles (14.5953, 10.4743) (14.6842, 10.3496) (14.8834, 10.2277) (15.0074, 10.2069) knots 0 0 0 1 2 2 2
  spline S171 degree 2 poles (15.0074, 10.2069) (15.132, 10.1896) (15.3626, 10.2449) (15.4885, 10.3194) knots 0 0 0 1 2 2 2
  line L167 (15.4885, 10.3194) -> (14.7871, 11.3028)
  line L168 (12.5524, 12.5396) -> (14.8345, 13.4151)
  line L169 (14.8345, 13.4151) -> (15.0643, 13.1567)
  line L170 (15.0643, 13.1567) -> (13.9228, 10.9983)
  line L171 (13.9228, 10.9983) -> (13.6454, 11.3102)
  line L172 (13.6454, 11.3102) -> (14.5464, 12.9474)
  line L173 (14.5464, 12.9474) -> (12.8183, 12.2406)
  line L174 (12.8183, 12.2406) -> (12.5524, 12.5396)
  line L175 (11.7785, 16.1838) -> (12.9446, 15.2611)
  line L176 (12.9446, 15.2611) -> (12.7515, 15.0171)
  line L177 (12.7515, 15.0171) -> (12.3176, 15.3604)
  line L178 (12.3176, 15.3604) -> (11.0501, 13.7585)
  line L179 (11.0501, 13.7585) -> (11.484, 13.4152)
  line L180 (11.484, 13.4152) -> (11.3108, 13.1963)
  spline S172 degree 2 poles (11.3108, 13.1963) (11.0648, 13.3909) (10.722, 13.4354) (10.5532, 13.2539) knots 0 0 0 1 2 2 2
  line L181 (10.5532, 13.2539) -> (10.3053, 13.4501)
  line L182 (10.3053, 13.4501) -> (12.0096, 15.6041)
  line L183 (12.0096, 15.6041) -> (11.5854, 15.9397)
  line L184 (11.5854, 15.9397) -> (11.7785, 16.1838)
  line L185 (10.767, 16.8562) -> (11.1759, 16.588)
  line L186 (11.1759, 16.588) -> (10.8562, 16.1005)
  line L187 (10.8562, 16.1005) -> (10.4472, 16.3688)
  line L188 (10.4472, 16.3688) -> (10.767, 16.8562)
  spline S173 degree 2 poles (7.8626, 16.7479) (8.2498, 17.4708) (9.0327, 17.923) (9.4704, 17.6886) knots 0 0 0 1 2 2 2
  spline S174 degree 2 poles (9.4704, 17.6886) (9.9145, 17.4507) (9.9608, 16.5377) (9.5818, 15.83) knots 0 0 0 1 2 2 2
  spline S175 degree 2 poles (9.5818, 15.83) (9.1923, 15.1028) (8.4117, 14.655) (7.9719, 14.8906) knots 0 0 0 1 2 2 2
  spline S176 degree 2 poles (7.9719, 14.8906) (7.5299, 15.1273) (7.4871, 16.0468) (7.8626, 16.7479) knots 0 0 0 1 2 2 2
  spline S177 degree 2 poles (8.7627, 17.3194) (8.6393, 17.2146) (8.3765, 16.8286) (8.2284, 16.552) knots 0 0 0 1 2 2 2
  spline S178 degree 2 poles (8.2284, 16.552) (8.0803, 16.2755) (7.9058, 15.845) (7.8868, 15.6787) knots 0 0 0 1 2 2 2
  spline S179 degree 2 poles (7.8868, 15.6787) (7.8678, 15.5123) (7.9814, 15.2694) (8.1316, 15.1889) knots 0 0 0 1 2 2 2
  spline S180 degree 2 poles (8.1316, 15.1889) (8.2819, 15.1084) (8.5515, 15.1462) (8.6839, 15.2574) knots 0 0 0 1 2 2 2
  spline S181 degree 2 poles (8.6839, 15.2574) (8.8118, 15.3654) (9.0749, 15.7625) (9.216, 16.026) knots 0 0 0 1 2 2 2
  spline S182 degree 2 poles (9.216, 16.026) (9.3676, 16.309) (9.5356, 16.7065) (9.5583, 16.8849) knots 0 0 0 1 2 2 2
  spline S183 degree 2 poles (9.5583, 16.8849) (9.5807, 17.0523) (9.4674, 17.3063) (9.3106, 17.3903) knots 0 0 0 1 2 2 2
  spline S184 degree 2 poles (9.3106, 17.3903) (9.1625, 17.4696) (8.8929, 17.4318) (8.7627, 17.3194) knots 0 0 0 1 2 2 2
  point P0 (0, -18.25)
  dimension "d16" = 40
  constraints: 2 end point, 2 vertical alignment, 1 centre point, 1 coincident, 1 collinear, 1 midpoint, 1 vertical, 5 other
  measures "d16" diameter of A3
extrude "Wyciągnięcie proste2" add sketch "Szkic3" along normal blind 0.3 contours L109 L110 L111 L112 L113 L114 A3 L104 L105 L106 L0 | L0 A3 L108 L109 | A3 L106 L107 L0 | L0 L107 L108 A3 | S173 S174 A3 | A3 S174 S175 S176 S173 | L3 L4 S2 S3 S0 S1 A3 | A3 S1 L2 L3 | S126 S110 A3 | A3 S110 L99 L100 S111 S112 S113 S114 S115 S116 S117 S118 S119 L101 L102 S120 S121 S122 S123 S124 S125 S126 | A3 L114 L103 L104 | A3 L186 L187 L188 | S8 S9 S10 S11 L8 L9 S12 S13 S14 L10 L11 S15 S16 A3 | A3 S16 S8 | L98 L91 L92 A3 | A3 L92 S104 S105 S106 L93 L94 L95 S107 S108 S109 L96 L97 L98 | S128 S129 S130 S127 A3 | A3 S127 S128 | L184 L175 A3 | A3 L176 L177 L178 L179 L180 S172 L181 L182 L183 L184 | S21 L13 L14 S22 S23 S24 S25 S26 S27 S28 S29 S30 L15 L16 S31 S32 S33 S34 S35 S36 S37 A3 | A3 S37 S21 | L175 L176 A3 | S104 S105 A3 | L120 L121 L122 L123 L124 L125 L126 L127 L115 A3 L117 L118 | A3 L118 L119 L120 | L18 L19 L20 A3 | A3 L170 L171 L172 L173 L174 L168 | L90 L79 L80 A3 | A3 L80 L81 L82 L84 L85 L86 L87 L88 L89 L90 | A3 L115 L116 L117 | S41 L25 S42 S43 S44 S45 S46 L26 L27 L28 S47 A3 | A3 S47 S48 L29 L30 S38 S39 S40 S41 | S167 S159 A3 | A3 S159 S160 S161 S162 L163 L164 S163 S164 S165 L165 L166 S166 S167 | L82 L83 L84 A3 | S135 L128 L129 S136 S137 S138 S139 S140 S141 S142 S143 S144 L130 L131 S145 S146 S147 S148 S149 S150 S151 A3 | A3 S151 S135 | L36 L37 L38 S56 S57 L39 A3 L33 S53 S54 S55 L34 | A3 L34 L35 L36 | L159 L152 L153 A3 | A3 L153 L154 L155 L157 L158 S152 S153 S154 L159 | A3 L76 L77 L78 | L137 L138 L139 L140 L141 L142 L143 A3 L133 L134 L135 | A3 L135 L136 L137 | A3 L39 L32 L33 | L155 L156 L157 A3 | L65 L66 A3 | A3 L66 L67 S92 S93 S94 L68 S95 S90 S91 | A3 L143 L132 L133 | S58 S59 S60 S61 L40 L41 S62 S63 S64 L42 L43 S65 S66 A3 | A3 S66 S58 | L57 L58 L59 A3 | A3 L59 L60 L61 L62 L63 L64 L57 | L145 L146 L147 A3 | S73 S74 S75 S76 S77 L47 L48 L49 A3 L46 S71 S72 | A3 S72 S73 | S82 S83 A3 | A3 S83 L51 L53 L54 L55 S84 S85 S82 | A3 L49 L45 L46 | L51 L52 L53 A3 | L21 L22 L23 L24 | L148 L149 L150 L151
equation "\"d13\" = name_plate_d"
equation "\"d14\" = name_plate_D"
equation "\"d15\" = name_plate_insert_r"
equation "\"d6\" = insert_m2_pocket_d"
equation "\"d8\" = insert_m2_pocket_D"
equation "\"d9\" = insert_m2_pocket_nut_h"
equation "\"d16\" = name_plate_text_d"
equation "\"insert_m2_d\" = 2.9"
equation "\"insert_m2_h\" = 7"
equation "\"insert_m2_corner\" = 0.5"
equation "\"insert_m2_pocket_d\" = 2.6"
equation "\"insert_m2_pocket_D\" = 4.5"
equation "\"insert_m2_pocket_nut_h\" = 1.5"
equation "\"stator_r_out\" = 30.15"
equation "\"stator_out_d\" = 3.2"
equation "\"stator_h\" = 45"
equation "\"stator_radial_screw_d\" = 4"
equation "\"stator_radial_screw_pos\" = 4"
equation "\"mag_size_x\" = 7"
equation "\"mag_size_y\" = 3"
equation "\"mag_corner_r\" = 0.4"
equation "\"magnet_ring_r\" = 26.95"
equation "\"magnet_ring_d\" = 3.3"
equation "\"magnet_ring_h\" = 36"
equation "\"magnet_ring_pocket_mag_size_x\" = 7.1"
equation "\"magnet_ring_pocket_mag_size_y\" = 3.1"
equation "\"magnet_ring_pocket_mag_size_z\" = 10.1"
equation "\"magnet_ring_pocket_radial_cut\" = 1.4"
equation "\"magnet_ring_insert_part_lengthen\" = 8"
equation "\"magnet_ring_insert_part_axial_flat_cut\" = 0.17"
equation "\"magnet_ring_insert_pos\" = 4"
equation "\"casing_d\" = 3"
equation "\"casing_r_in\" = 30.15"
equation "\"casing_lock_hole_r\" = 14.25"
equation "\"casing_lock_h\" = 8"
equation "\"casing_stator_fix_r\" = 23"
equation "\"casing_stator_fix_h\" = 6"
equation "\"casing_sidebar_length\" = 3"
equation "\"casing_vent_hole_length\" = 4"
equation "\"casing_vent_hole_width\" = 6"
equation "\"casing_head_insert_r\" = 19"
equation "\"casing_radial_stator_insert_pos\" = 18.1"
equation "\"casing_cart_hole_ang\" = 90deg"
equation "\"casing_cart_hole_width\" = 2.6"
equation "\"casing_cart_hole_corner\" = 1"
equation "\"casing_cart_hole_pos\" = 17"
equation "\"casing_sleeve_cut_d\" = 46"
equation "\"casing_sleeve_cut_h\" = 4"
equation "\"casing_backsleeve_insert_pos\" = 4.9"
equation "\"rotor_out_r\" = 22.5"
equation "\"rotor_coil_groove_in_r\" = 17"
equation "\"rotor_coil_groove_ang\" = 18deg"
equation "\"rotor_core_r\" = 14.97"
equation "\"rotor_coil_groove_in_correction_r\" = 18"
equation "\"rotor_plastic_h\" = 32"
equation "\"rotor_teeth_d\" = 1.5"
equation "\"rotor_plastic_insert_r\" = 37"
equation "\"shaft_d\" = 8"
equation "\"shaft_lock_1_d\" = 8.1"
equation "\"shaft_lock_1_D\" = 44"
equation "\"shaft_lock_1_h1\" = 3.5"
equation "\"shaft_lock_1_corner\" = 2"
equation "\"shaft_lock_1_rotor_insert_grove_d_in\" = 36"
equation "\"shaft_lock_1_rotor_insert_grove_width_out\" = 5.5"
equation "\"shaft_lock_1_rotor_insert_grove_width_in\" = 7.6"
equation "\"shaft_lock_1_rotor_insert_r\" = 37"
equation "\"shaft_lock_1_shaft_insert_axial_cut_out_width\" = 12"
equation "\"shaft_lock_1_shaft_insert_axial_cut_in_width\" = 5.4"
equation "\"shaft_lock_1_shaft_insert_pos\" = 2.5"
equation "\"shaft_lock_1_shaft_insert_corner\" = 2"
equation "\"shaft_lock_1_shaft_insert_corner_finish\" = 0.5"
equation "\"shaft_lock_2_d\" = 8.1"
equation "\"shaft_lock_2_D\" = 44"
equation "\"shaft_lock_2_h1\" = 3.5"
equation "\"shaft_lock_2_corner\" = 2"
equation "\"shaft_lock_2_rotor_insert_grove_d_in\" = 36"
equation "\"shaft_lock_2_rotor_insert_grove_width_out\" = 5.5"
equation "\"shaft_lock_2_rotor_insert_grove_width_in\" = 7.6"
equation "\"shaft_lock_2_rotor_insert_r\" = 37"
equation "\"shaft_lock_2_shaft_insert_axial_cut_out_width\" = 12"
equation "\"shaft_lock_2_shaft_insert_axial_cut_in_width\" = 5.4"
equation "\"shaft_lock_2_shaft_insert_pos\" = 2.5"
equation "\"shaft_lock_2_shaft_insert_corner\" = 2"
equation "\"shaft_lock_2_shaft_insert_corner_finish\" = 0.5"
equation "\"commutator_plastic_shaft_d\" = 8.1"
equation "\"commutator_plastic_h\" = 17"
equation "\"commutator_plastic_insert_cut_deepness\" = 0.5"
equation "\"commutator_plastic_insert_cut_length\" = 6"
equation "\"commutator_plastic_insert_pos\" = 3"
equation "\"commutator_plate_D\" = 22"
equation "\"commutator_plate_d\" = 1"
equation "\"commutator_plate_ang\" = 55deg"
equation "\"commutator_plate_h\" = 17"
equation "\"commutator_plate_insert_pos\" = 3"
equation "\"sleeve_in_r\" = 11.1"
equation "\"sleeve_d\" = 3"
equation "\"sleeve_h\" = 7"
equation "\"sleeve_cup_r\" = 22"
equation "\"sleeve_cup_h\" = 4.5"
equation "\"sleeve_head_insert_r\" = 19"
equation "\"rotor_sleeve_in_D\" = 8.15"
equation "\"rotor_sleeve_out_D\" = 10.5"
equation "\"rotor_sleeve_h\" = 32"
equation "\"carbon_brush_batt_d\" = 4"
equation "\"carbon_brush_batt_h\" = 8"
equation "\"brush_cart_outer_holder_width\" = 5.5"
equation "\"brush_cart_outer_holder_arc_r\" = 33.15"
equation "\"brush_cart_outer_holder_arc_pos\" = 1.5"
equation "\"brush_holder_batt_width\" = 16"
equation "\"brush_holder_batt_arc_r\" = 30.15"
equation "\"brush_holder_batt_insert_flat_length\" = 6"
equation "\"brush_holder_batt_insert_flat_depth\" = 6"
equation "\"brush_holder_batt_brush_hole_d\" = 4.5"
equation "\"name_plate_D\" = 45"
equation "\"name_plate_d\" = 28"
equation "\"name_plate_insert_r\" = 19"
equation "\"name_plate_text_d\" = 40"
equation "\"sleeve_bearing_material_lock_h\" = 2"
equation "\"back_sleeve_D\" = 66"
equation "\"back_sleeve_d\" = 22.2"
equation "\"back_sleeve_h\" = 5"
equation "\"commutator_back_plate_lock_h\" = 2"
equation "\"commutator_back_plate_lock_r\" = 23"
equation "\"commutator_plastic_back_plate_lock_r\" = 11.9"
equation "\"commutator_plastic_back_plate_lock_h\" = 1"
equation "\"commutator_plastic_back_plate_hook_in_r\" = 11.15"
equation "\"commutator_plastic_back_plate_hook_d\" = 1"
